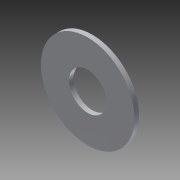
# Autodesk Inventor part: 01
Saved by Autodesk Inventor 2013 (Build 170138000, 138)
## iProperties
Created: 2014-02-13
Material: アセタール樹脂、白
Document SubType Name: Modeling
Designer: andou
Density: 1.425 g/cm^3
Mass: 0.376049 g
Surface Area: 6.15752 cm^2
Volume: 0.263894 cm^3
Part Number: 01
Author: andou
Title: Acetal_Washer
Autodesk Inventor part; units mm, degrees
ref_plane "YZ Plane" through (0, 0, 0) normal (1, 0, 0) x (0, 1, 0)
ref_plane "XZ Plane" through (0, 0, 0) normal (0, 1, 0) x (-1, 0, 0)
ref_plane "XY Plane" through (0, 0, 0) normal (0, 0, 1) x (1, 0, 0)
sketch "スケッチ1" plane through (0, 0, 0) normal (0, 1, 0) x (-1, 0, 0)
  circle A0 centre (0, 0) radius 10
  circle A1 centre (0, 0) radius 4
  dimension "d0" = 20
  dimension "d2" = 8
  constraints: 2 centre point, 2 coincident
  measures "d0" diameter of A0
  measures "d2" diameter of A1
extrude "押し出し1" add sketch "スケッチ1" along normal blind 1
